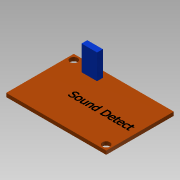
# Autodesk Inventor part: Sound Detect
Saved by Autodesk Inventor 2015 SP1 (Build 190203100, 203)
## iProperties
Created: 2015-01-28
Part Number: Sound Detect
Material: Generic
Document SubType Name: Modeling
Designer: Rafi Kurnia Putra
Density: 1 g/cm^3
Appearance: Smooth - Light Orange
Author: Rafi Kurnia Putra
Autodesk Inventor part; units mm, degrees
ref_plane "YZ Plane" through (0, 0, 0) normal (1, 0, 0) x (0, 1, 0)
ref_plane "XZ Plane" through (0, 0, 0) normal (0, 1, 0) x (-1, 0, 0)
ref_plane "XY Plane" through (0, 0, 0) normal (0, 0, 1) x (1, 0, 0)
sketch "Sketch1" plane through (0, 0, 0) normal (0, 1, 0) x (-1, 0, 0)
  line L0 (23.25, 15.71) -> (-23.25, 15.71)
  line L1 (-23.25, 15.71) -> (-23.25, -15.71)
  line L2 (-23.25, -15.71) -> (23.25, -15.71)
  line L3 (23.25, -15.71) -> (23.25, 15.71)
  line L4 (23.25, 15.71) -> (-23.25, -15.71) construction
  line L5 (-23.25, 15.71) -> (23.25, -15.71) construction
  circle A0 centre (20.75, -13.21) radius 1.75
  circle A1 centre (-20.75, 13.21) radius 1.75
  line L6 (14.0587, -12.8063) -> (6.8338, -12.8063)
  line L7 (6.8338, -12.8063) -> (6.8338, -10.1137)
  line L8 (6.8338, -10.1137) -> (14.0587, -10.1137)
  line L9 (14.0587, -10.1137) -> (14.0587, -12.8063)
  line L10 (14.0587, -12.8063) -> (6.8338, -10.1137) construction
  line L11 (6.8338, -12.8063) -> (14.0587, -10.1137) construction
  point P0 (0, 0)
  point P1 (10.4463, -11.46)
  dimension "d0" = 46.5
  dimension "d1" = 31.42
  dimension "d2" = 3.5
  dimension "d3" = 3.5
  dimension "d4" = 2.5
  dimension "d5" = 2.5
  dimension "d6" = 2.5
  dimension "d7" = 2.5
  constraints: 24 end point, 4 midpoint, 4 parallel, 2 centre point, 2 horizontal, 2 perpendicular
  measures "d0" distance of L2.end L1.end
  measures "d1" distance of L1.end L0.end
  measures "d2" diameter of A0
  measures "d3" diameter of A1
  measures "d4" distance from line of L3 A0.centre
  measures "d5" distance from line of L2 A0.centre
  measures "d6" distance from line of L1 A1.centre
  measures "d7" distance from line of L0 A1.centre
extrude "Extrusion1" add sketch "Sketch1" along normal blind 1.7
extrude "Extrusion2" add sketch "Sketch1" along normal blind 13.25 contours L6 L7 L8 L9
sketch "Sketch2" plane through (0, 1.7, 0) normal (0, 1, 0) x (1, 0, 0)
  line L0 (-8.2019, 1.2171) -> (20.3938, 1.2171) construction
  line L1 (20.3938, 1.2171) -> (20.3938, -2.5127) construction
  line L2 (20.3938, -2.5127) -> (-8.2019, -2.5127) construction
  line L3 (-8.2019, -2.5127) -> (-8.2019, 1.2171) construction
  point P0 (0, 0)
  constraints: 2 other
sketch "Sketch3" plane through (23.25, 0, -15.71) normal (0, 0, -1) x (-1, 0, 0)
  point P0 (23.25, 0)
body "Solid1"
